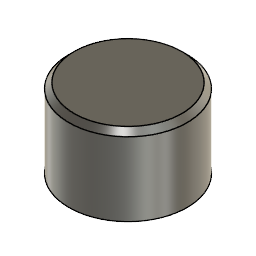
LeftLegJoint (Autodesk Fusion 360 archive; units mm, degrees)
design "Cap"
Autodesk Fusion 360 part; units mm, degrees
sketch "Sketch1" plane through (0, 0, 0) normal (0, 0, 1) x (1, 0, 0)
  circle A0 centre (0, 0) radius 2.25
  line L0 (0, -2.25) -> (0, 2.25) construction
  circle A1 centre (0, 0) radius 2.05
  line L1 (-2.8, 0) -> (3.3, 0) construction
  line L2 (-0.3101, 1.2109) -> (-0.3806, 1.3992)
  line L3 (-0.3101, -1.2109) -> (-0.3806, -1.3992)
  line L4 (0.3101, 1.2109) -> (0.3806, 1.3992)
  line L5 (0.3101, -1.2109) -> (0.3806, -1.3992)
  arc A2 (0.3101, -1.2109) -> (0.3101, 1.2109) centre (0, 0) ccw
  arc A3 (-0.3101, 1.2109) -> (-0.3101, -1.2109) centre (0, 0) ccw
  arc A4 (0.3806, -1.3992) -> (0.3806, 1.3992) centre (0, 0) ccw
  arc A5 (-0.3806, 1.3992) -> (-0.3806, -1.3992) centre (0, 0) ccw
  spline S0 degree 5 poles (-0.6611, 1.2905) (-0.6844, 1.2837) (-0.7307, 1.2707) (-0.7989, 1.2529) (-0.8873, 1.2327) (-0.9934, 1.2139) (-1.0947, 1.2022) (-1.1908, 1.198) (-1.2813, 1.2018) (-1.3665, 1.2133) (-1.4468, 1.2321) (-1.5073, 1.2524) (-1.5508, 1.2704) (-1.5789, 1.2836) (-1.5928, 1.2905) knots 0 0 0 0 0 0 0.1 0.2 0.3 0.4 0.5 0.6 0.7 0.8 0.9 1 1 1 1 1 1
  spline S1 degree 5 poles (-1.1074, 0.936) (-1.124, 0.9409) (-1.1571, 0.9501) (-1.206, 0.9627) (-1.2701, 0.977) (-1.348, 0.9902) (-1.4235, 0.9985) (-1.4965, 1.0014) (-1.5669, 0.9987) (-1.6346, 0.9905) (-1.7, 0.9772) (-1.7506, 0.9629) (-1.7876, 0.9502) (-1.8118, 0.9409) (-1.8238, 0.936) knots 0 0 0 0 0 0 0.1 0.2 0.3 0.4 0.5 0.6 0.7 0.8 0.9 1 1 1 1 1 1
  spline S2 degree 5 poles (-1.1074, -0.936) (-1.124, -0.9409) (-1.1571, -0.9501) (-1.206, -0.9627) (-1.2701, -0.977) (-1.348, -0.9902) (-1.4235, -0.9985) (-1.4965, -1.0014) (-1.5669, -0.9987) (-1.6346, -0.9905) (-1.7, -0.9772) (-1.7506, -0.9629) (-1.7876, -0.9502) (-1.8118, -0.9409) (-1.8238, -0.936) knots 0 0 0 0 0 0 0.1 0.2 0.3 0.4 0.5 0.6 0.7 0.8 0.9 1 1 1 1 1 1
  line L6 (-1.0301, 0.9135) -> (-1.1847, 0.9585)
  line L7 (-1.7583, 0.9626) -> (-1.8894, 0.9095)
  line L8 (-1.0301, -0.9135) -> (-1.1847, -0.9585)
  line L9 (-1.7583, -0.9626) -> (-1.8894, -0.9095)
  spline S3 degree 5 poles (-0.6611, -1.2905) (-0.6844, -1.2837) (-0.7307, -1.2707) (-0.7989, -1.2529) (-0.8873, -1.2327) (-0.9934, -1.2139) (-1.0947, -1.2022) (-1.1908, -1.198) (-1.2813, -1.2018) (-1.3665, -1.2133) (-1.4468, -1.2321) (-1.5073, -1.2524) (-1.5508, -1.2704) (-1.5789, -1.2836) (-1.5928, -1.2905) knots 0 0 0 0 0 0 0.1 0.2 0.3 0.4 0.5 0.6 0.7 0.8 0.9 1 1 1 1 1 1
  line L10 (-0.5569, 1.321) -> (-0.7652, 1.2601)
  line L11 (-1.5135, 1.2509) -> (-1.6721, 1.3301)
  line L12 (-0.5569, -1.321) -> (-0.7652, -1.2601)
  line L13 (-1.5135, -1.2509) -> (-1.6721, -1.3301)
  spline S4 degree 5 poles (0.6611, -1.2905) (0.6844, -1.2837) (0.7307, -1.2707) (0.7989, -1.2529) (0.8873, -1.2327) (0.9934, -1.2139) (1.0947, -1.2022) (1.1908, -1.198) (1.2813, -1.2018) (1.3665, -1.2133) (1.4468, -1.2321) (1.5073, -1.2524) (1.5508, -1.2704) (1.5789, -1.2836) (1.5928, -1.2905) knots 0 0 0 0 0 0 0.1 0.2 0.3 0.4 0.5 0.6 0.7 0.8 0.9 1 1 1 1 1 1
  line L14 (0.5569, -1.321) -> (0.7652, -1.2601)
  line L15 (1.5135, -1.2509) -> (1.6721, -1.3301)
  spline S5 degree 5 poles (1.1074, -0.936) (1.124, -0.9409) (1.1571, -0.9501) (1.206, -0.9627) (1.2701, -0.977) (1.348, -0.9902) (1.4235, -0.9985) (1.4965, -1.0014) (1.5669, -0.9987) (1.6346, -0.9905) (1.7, -0.9772) (1.7506, -0.9629) (1.7876, -0.9502) (1.8118, -0.9409) (1.8238, -0.936) knots 0 0 0 0 0 0 0.1 0.2 0.3 0.4 0.5 0.6 0.7 0.8 0.9 1 1 1 1 1 1
  line L16 (1.0301, -0.9135) -> (1.1847, -0.9585)
  line L17 (1.7583, -0.9626) -> (1.8894, -0.9095)
  spline S6 degree 5 poles (1.1074, 0.936) (1.124, 0.9409) (1.1571, 0.9501) (1.206, 0.9627) (1.2701, 0.977) (1.348, 0.9902) (1.4235, 0.9985) (1.4965, 1.0014) (1.5669, 0.9987) (1.6346, 0.9905) (1.7, 0.9772) (1.7506, 0.9629) (1.7876, 0.9502) (1.8118, 0.9409) (1.8238, 0.936) knots 0 0 0 0 0 0 0.1 0.2 0.3 0.4 0.5 0.6 0.7 0.8 0.9 1 1 1 1 1 1
  line L18 (1.0301, 0.9135) -> (1.1847, 0.9585)
  line L19 (1.7583, 0.9626) -> (1.8894, 0.9095)
  spline S7 degree 5 poles (0.6611, 1.2905) (0.6844, 1.2837) (0.7307, 1.2707) (0.7989, 1.2529) (0.8873, 1.2327) (0.9934, 1.2139) (1.0947, 1.2022) (1.1908, 1.198) (1.2813, 1.2018) (1.3665, 1.2133) (1.4468, 1.2321) (1.5073, 1.2524) (1.5508, 1.2704) (1.5789, 1.2836) (1.5928, 1.2905) knots 0 0 0 0 0 0 0.1 0.2 0.3 0.4 0.5 0.6 0.7 0.8 0.9 1 1 1 1 1 1
  line L20 (0.5569, 1.321) -> (0.7652, 1.2601)
  line L21 (1.5135, 1.2509) -> (1.6721, 1.3301)
  point P0 (-1.2, 1.2)
  point P1 (-1.5, 1)
  point P2 (-1.5, -1)
  point P3 (-1.2, -1.2)
  point P4 (1.2, -1.2)
  point P5 (1.5, -1)
  point P6 (1.5, 1)
  point P7 (1.2, 1.2)
  dimension "d1" = 4.5
  dimension "d2" = 2.5
  dimension "d4" = -0.2
  constraint coincident A0.centre A1.centre
  constraint concentric A0 A2
  constraint coincident A0 L0.start
  constraint coincident A0 L0.end
  constraint vertical L0
  constraint horizontal L1
  constraint symmetric L1 L2.start L3.start
  constraint symmetric L1 L2.end L3.end
  constraint symmetric L0 L2.start L4.start
  constraint symmetric L0 L3.start L5.start
  constraint concentric A2 A4
  constraint concentric A2 A3
  constraint concentric A4 A5
  constraint coincident A5 S0.start
  constraint coincident A1 S0.end
  constraint coincident A5 S1.start
  constraint coincident A1 S1.end
  constraint midpoint S1.start L6
  constraint midpoint S1.end L7
  constraint midpoint S0.start L10
  constraint midpoint S0.end L11
  constraint symmetric L1 S0.start S3.start
  constraint symmetric L1 P0 P3
  constraint symmetric L1 S0.end S3.end
  constraint symmetric L1 S1.start S2.start
  constraint symmetric L1 P1 P2
  constraint symmetric L1 S1.end S2.end
  constraint symmetric L1 L6.start L8.start
  constraint symmetric L1 L6.end L8.end
  constraint symmetric L1 L7.start L9.start
  constraint symmetric L1 L7.end L9.end
  constraint symmetric L1 L10.start L12.start
  constraint symmetric L1 L10.end L12.end
  constraint symmetric L1 L11.start L13.start
  constraint symmetric L1 L11.end L13.end
  constraint symmetric L0 S0.start S7.start
  constraint symmetric L0 P0 P7
  constraint symmetric L0 S0.end S7.end
  constraint symmetric L0 S1.start S6.start
  constraint symmetric L0 P1 P6
  constraint symmetric L0 S1.end S6.end
  constraint symmetric L0 S2.start S5.start
  constraint symmetric L0 P2 P5
  constraint symmetric L0 S2.end S5.end
  constraint symmetric L0 L6.start L18.start
  constraint symmetric L0 L6.end L18.end
  constraint symmetric L0 L7.start L19.start
  constraint symmetric L0 L7.end L19.end
  constraint symmetric L0 L8.start L16.start
  constraint symmetric L0 L8.end L16.end
  constraint symmetric L0 L9.start L17.start
  constraint symmetric L0 L9.end L17.end
  constraint symmetric L0 S3.start S4.start
  constraint symmetric L0 P3 P4
  constraint symmetric L0 S3.end S4.end
  constraint symmetric L0 L10.start L20.start
  constraint symmetric L0 L10.end L20.end
  constraint symmetric L0 L11.start L21.start
  constraint symmetric L0 L11.end L21.end
  constraint symmetric L0 L12.start L14.start
  constraint symmetric L0 L12.end L14.end
  constraint symmetric L0 L13.start L15.start
  constraint symmetric L0 L13.end L15.end
  measures "d1" diameter of A0
  measures "d2" diameter of A2
extrude "Extrude1" add sketch "Sketch1" along normal blind 2 contours A0 | A1 A4 S6 L18 S7 L20 | A1 A5 S0 S1 L6 L10 | L4 L5 A2 A4 | A1 A5 S2 L8 S3 L12 | L2 L3 A3 A5
extrude "Extrude2" add sketch "Sketch1" along normal blind 1 from surface at 2 contours A0 | A1 A4 S5 L16 S6 L18 | A1 A4 S6 L18 S7 L20 | A1 A4 S4 L14 S5 L16 | A1 L2 L3 L4 L5 A2 A3 A4 A5 S0 S3 L10 L12 S4 L14 S7 L20 | A1 A5 S0 S1 L6 L10 | L4 L5 A2 A4 | A1 A5 S2 L8 S3 L12 | A1 A5 S1 S2 L6 L8 | L2 L3 A3 A5
chamfer "Chamfer1" distance 0.2 angle 45 1 edges at (-2.0977, -0.8136, 3)
extrude "Extrude3" add sketch "Sketch1" along normal blind 2 contours A1 A4 S4 S5
